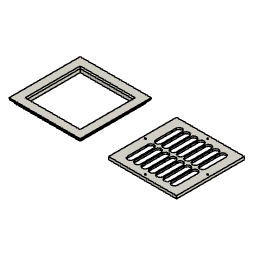
Magneto+Filter+Lüfter (Autodesk Fusion 360 design; units mm, degrees)
Autodesk Fusion 360 part; units mm, degrees
sketch "Skizze1" plane through (0, 0, 0) normal (0, 0, 1) x (1, 0, 0)
  line L0 (173.376542, 106.779405) -> (293.376542, 106.779405)
  line L1 (293.376542, 106.779405) -> (293.376542, -13.220595)
  line L2 (293.376542, -13.220595) -> (173.376542, -13.220595)
  line L3 (173.376542, -13.220595) -> (173.376542, 106.779405)
  line L4 (283.376542, -3.220595) -> (183.376542, -3.220595)
  line L5 (183.376542, -3.220595) -> (183.376542, 96.779405)
  line L6 (183.376542, 96.779405) -> (283.376542, 96.779405)
  line L7 (283.376542, 96.779405) -> (283.376542, -3.220595)
  line L8 (286.376542, -6.220595) -> (180.376542, -6.220595)
  line L9 (180.376542, -6.220595) -> (180.376542, 99.779405)
  line L10 (180.376542, 99.779405) -> (286.376542, 99.779405)
  line L11 (286.376542, 99.779405) -> (286.376542, -6.220595)
  circle A0 centre (233.376542, 103.279405) radius 1.5
  circle A1 centre (289.876542, 46.779405) radius 1.5
  circle A2 centre (176.876542, 46.779405) radius 1.5
  circle A3 centre (233.376542, -9.720595) radius 1.5
  circle A4 centre (423.376542, 103.279405) radius 1.5
  line L12 (483.376542, 106.779405) -> (483.376542, -13.220595)
  circle A5 centre (479.876542, 46.779405) radius 1.5
  line L13 (363.376542, 106.779405) -> (483.376542, 106.779405)
  circle A6 centre (366.876542, 46.779405) radius 1.5
  line L14 (363.376542, -13.220595) -> (363.376542, 106.779405)
  circle A7 centre (423.376542, -9.720595) radius 1.5
  line L15 (483.376542, -13.220595) -> (363.376542, -13.220595)
  line L16 (469.376542, 90.779405) -> (469.376542, 2.779405)
  line L17 (458.376542, 90.779405) -> (458.376542, 2.779405)
  arc A8 (469.376542, 90.779405) -> (458.376542, 90.779405) centre (463.876542, 90.779405) ccw
  arc A9 (458.376542, 2.779405) -> (469.376542, 2.779405) centre (463.876542, 2.779405) ccw
  line L18 (456.043208, 90.779405) -> (456.043208, 2.779405)
  arc A10 (456.043208, 90.779405) -> (445.043208, 90.779405) centre (450.543208, 90.779405) ccw
  line L19 (445.043208, 90.779405) -> (445.043208, 2.779405)
  arc A11 (445.043208, 2.779405) -> (456.043208, 2.779405) centre (450.543208, 2.779405) ccw
  line L20 (442.709875, 90.779405) -> (442.709875, 2.779405)
  arc A12 (442.709875, 90.779405) -> (431.709875, 90.779405) centre (437.209875, 90.779405) ccw
  line L21 (431.709875, 90.779405) -> (431.709875, 2.779405)
  arc A13 (431.709875, 2.779405) -> (442.709875, 2.779405) centre (437.209875, 2.779405) ccw
  line L22 (429.376542, 90.779405) -> (429.376542, 2.779405)
  arc A14 (429.376542, 90.779405) -> (418.376542, 90.779405) centre (423.876542, 90.779405) ccw
  line L23 (418.376542, 90.779405) -> (418.376542, 2.779405)
  arc A15 (418.376542, 2.779405) -> (429.376542, 2.779405) centre (423.876542, 2.779405) ccw
  line L24 (416.043208, 90.779405) -> (416.043208, 2.779405)
  arc A16 (416.043208, 90.779405) -> (405.043208, 90.779405) centre (410.543208, 90.779405) ccw
  line L25 (405.043208, 90.779405) -> (405.043208, 2.779405)
  arc A17 (405.043208, 2.779405) -> (416.043208, 2.779405) centre (410.543208, 2.779405) ccw
  line L26 (402.709875, 90.779405) -> (402.709875, 2.779405)
  arc A18 (402.709875, 90.779405) -> (391.709875, 90.779405) centre (397.209875, 90.779405) ccw
  line L27 (391.709875, 90.779405) -> (391.709875, 2.779405)
  arc A19 (391.709875, 2.779405) -> (402.709875, 2.779405) centre (397.209875, 2.779405) ccw
  line L28 (389.376542, 90.779405) -> (389.376542, 2.779405)
  arc A20 (389.376542, 90.779405) -> (378.376542, 90.779405) centre (383.876542, 90.779405) ccw
  line L29 (378.376542, 90.779405) -> (378.376542, 2.779405)
  arc A21 (378.376542, 2.779405) -> (389.376542, 2.779405) centre (383.876542, 2.779405) ccw
  dimension "d18" = 120
  dimension "d19" = 120
  dimension "d20" = 10
  dimension "d21" = 7
  dimension "d22" = 3
  dimension "d23" = 3
  dimension "d24" = 3
  dimension "d25" = 3
  dimension "d28" = 120
  dimension "d29" = 120
  dimension "d30" = 3
  dimension "d31" = 3
  dimension "d32" = 3
  dimension "d33" = 3
  dimension "d42" = -80
  dimension "d43" = 0
  constraint horizontal L0
  constraint vertical L1
  constraint horizontal L2
  constraint vertical L3
  constraint horizontal L13
  constraint vertical L12
  constraint horizontal L15
  constraint vertical L14
  constraint tangent L16 A9
  measures "d22" diameter of A0
  measures "d23" diameter of A1
  measures "d24" diameter of A2
  measures "d25" diameter of A3
  measures "d30" diameter of A4
  measures "d31" diameter of A5
  measures "d32" diameter of A6
  measures "d33" diameter of A7
extrude "Extrusion1" add sketch "Skizze1" along normal blind 10 contours L8 L9 L10 L11 picked at (216.709875, 98.779405) makes body 1
extrude "Extrusion2" add sketch "Skizze1" along normal blind 3 contours L0 L1 L2 L3 picked at (271.434124, -10.03234) bodies 1
extrude "Extrusion3" add sketch "Skizze1" along normal blind 3 separate body contours L12 L13 L14 L15 picked at (369.231464, 11.721823) makes body 2
sketch "Skizze2" plane through (0, 0, 10) normal (0, 0, 1) x (-1, 0, 0)
  line L0 (-183.376542, -96.779405) -> (-283.376542, -96.779405)
  line L1 (-283.376542, -96.779405) -> (-283.376542, 3.220595)
  line L2 (-283.376542, 3.220595) -> (-183.376542, 3.220595)
  line L3 (-183.376542, 3.220595) -> (-183.376542, -96.779405)
  line L4 (-286.376542, -99.779405) -> (-180.376542, -99.779405)
  line L5 (-180.376542, -99.779405) -> (-180.376542, 6.220595)
  line L6 (-180.376542, 6.220595) -> (-286.376542, 6.220595)
  line L7 (-286.376542, 6.220595) -> (-286.376542, -99.779405)
  line L8 (59.486834, 54.037754) -> (-90.513166, 54.037754)
  line L9 (-90.513166, 54.037754) -> (-90.513166, 204.037754)
  line L10 (-90.513166, 204.037754) -> (59.486834, 204.037754)
  line L11 (59.486834, 204.037754) -> (59.486834, 54.037754)
  line L12 (44.486834, 69.037754) -> (-75.513166, 69.037754)
  line L13 (-75.513166, 69.037754) -> (-75.513166, 189.037754)
  line L14 (-75.513166, 189.037754) -> (44.486834, 189.037754)
  line L15 (44.486834, 189.037754) -> (44.486834, 69.037754)
  dimension "d52" = 150
  dimension "d53" = 150
  dimension "d54" = 15
  constraint horizontal L8
  constraint vertical L9
  constraint horizontal L10
  constraint vertical L11
scale "Maßstab1" factor 1.2 about (283.376542, 96.779405, 0) bodies 1
scale "Maßstab2" factor 1.2 about (363.376542, 106.779405, 3) bodies 2
sketch "Skizze3" plane through (0, 0, 0) normal (0, 0, 1) x (1, 0, 0)
extrude "Extrusion4" add sketch "Skizze2" along normal blind 3 separate body contours L8 L9 L10 L11 picked at (-85.513166, 149.037754) makes body 3
move_body "Verschieben1" bodies 3 to x (1, 0, 0) y (0, 1, 0) z (0, 0, 1) at (207.863376, 165.817159, 2)
move_body "Verschieben2" bodies 3 to x (1, 0, 0) y (0, 1, 0) z (0, 0, 1) at (0, 0, -3)
move_body "Verschieben3" bodies 3 to x (1, 0, 0) y (0, 1, 0) z (0, 0, 1) at (0, 0, -1)
move_body "Verschieben4" bodies 3 to x (1, 0, 0) y (0, 1, 0) z (0, 0, 1) at (0, 0, -1)
extrude "Extrusion5" cut 1 faces at (203.376542, 99.179405, 12) along direction (0, 0, -1) blind 1 on bodies 1 bodies 1
extrude "Extrusion6" cut 1 faces at (203.376542, 99.179405, 11) along direction (0, 0, -1) blind 1 on bodies 1 bodies 1
combine "Kombinieren1" operation add target body 3 tool bodies 1
extrude "Extrusion7" add 1 faces at (155.202448, -8.889694, 3.6) along direction (0, 0, 1) blind 3.5 on bodies 3 bodies 3
sketch "Skizze4" plane through (0, 0, 3) normal (0, 0, 1) x (-1, 0, 0)
  arc A0 (-394.576542, -87.579405) -> (-381.376542, -87.579405) centre (-387.976542, -87.579405) ccw
  line L0 (-394.576542, -87.579405) -> (-394.576542, 18.020595)
  arc A1 (-381.376542, 18.020595) -> (-394.576542, 18.020595) centre (-387.976542, 18.020595) ccw
  line L1 (-381.376542, 18.020595) -> (-381.376542, -87.579405)
  circle A2 centre (-435.376542, 33.020595) radius 1.8
  arc A3 (-458.576542, -87.579405) -> (-445.376542, -87.579405) centre (-451.976542, -87.579405) ccw
  line L2 (-458.576542, -87.579405) -> (-458.576542, 18.020595)
  arc A4 (-445.376542, 18.020595) -> (-458.576542, 18.020595) centre (-451.976542, 18.020595) ccw
  line L3 (-445.376542, 18.020595) -> (-445.376542, -87.579405)
  arc A5 (-474.576542, -87.579405) -> (-461.376542, -87.579405) centre (-467.976542, -87.579405) ccw
  line L4 (-474.576542, -87.579405) -> (-474.576542, 18.020595)
  arc A6 (-461.376542, 18.020595) -> (-474.576542, 18.020595) centre (-467.976542, 18.020595) ccw
  line L5 (-461.376542, 18.020595) -> (-461.376542, -87.579405)
  arc A7 (-426.576542, -87.579405) -> (-413.376542, -87.579405) centre (-419.976542, -87.579405) ccw
  line L6 (-426.576542, -87.579405) -> (-426.576542, 18.020595)
  arc A8 (-413.376542, 18.020595) -> (-426.576542, 18.020595) centre (-419.976542, 18.020595) ccw
  line L7 (-413.376542, 18.020595) -> (-413.376542, -87.579405)
  circle A9 centre (-503.176542, -34.779405) radius 1.8
  arc A10 (-490.576542, -87.579405) -> (-477.376542, -87.579405) centre (-483.976542, -87.579405) ccw
  line L8 (-490.576542, -87.579405) -> (-490.576542, 18.020595)
  arc A11 (-477.376542, 18.020595) -> (-490.576542, 18.020595) centre (-483.976542, 18.020595) ccw
  line L9 (-477.376542, 18.020595) -> (-477.376542, -87.579405)
  arc A12 (-410.576542, -87.579405) -> (-397.376542, -87.579405) centre (-403.976542, -87.579405) ccw
  line L10 (-410.576542, -87.579405) -> (-410.576542, 18.020595)
  arc A13 (-397.376542, 18.020595) -> (-410.576542, 18.020595) centre (-403.976542, 18.020595) ccw
  line L11 (-397.376542, 18.020595) -> (-397.376542, -87.579405)
  circle A14 centre (-435.376542, -102.579405) radius 1.8
  circle A15 centre (-367.576542, -34.779405) radius 1.8
  arc A16 (-442.576542, -87.579405) -> (-429.376542, -87.579405) centre (-435.976542, -87.579405) ccw
  line L12 (-442.576542, -87.579405) -> (-442.576542, 18.020595)
  arc A17 (-429.376542, 18.020595) -> (-442.576542, 18.020595) centre (-435.976542, 18.020595) ccw
  line L13 (-429.376542, 18.020595) -> (-429.376542, -87.579405)
  line L14 (-507.376542, 37.220595) -> (-507.376542, -106.779405)
  line L15 (-507.376542, -106.779405) -> (-363.376542, -106.779405)
  line L16 (-363.376542, -106.779405) -> (-363.376542, 37.220595)
  line L17 (-363.376542, 37.220595) -> (-507.376542, 37.220595)
  line L18 (-509.376542, 39.220595) -> (-361.376542, 39.220595)
  line L19 (-361.376542, 39.220595) -> (-361.376542, -108.779405)
  line L20 (-361.376542, -108.779405) -> (-509.376542, -108.779405)
  line L21 (-509.376542, -108.779405) -> (-509.376542, 39.220595)
  line L22 (-363.376542, -106.779405) -> (-507.376542, -106.779405)
  line L23 (-507.376542, -106.779405) -> (-507.376542, 37.220595)
  line L24 (-507.376542, 37.220595) -> (-363.376542, 37.220595)
  line L25 (-363.376542, 37.220595) -> (-363.376542, -106.779405)
  constraint horizontal L18
  constraint vertical L19
  constraint horizontal L20
  constraint vertical L21
  constraint horizontal L22
  constraint vertical L23
  constraint horizontal L24
  constraint vertical L25
sketch "Skizze5" plane through (381.376542, 0, 0) normal (1, 0, 0) x (0, 1, 0)
  line L0 (-18.020595, -0.6) -> (87.579405, -0.6)
  line L1 (87.579405, -0.6) -> (87.579405, 3)
  line L2 (87.579405, 3) -> (-18.020595, 3)
  line L3 (-18.020595, 3) -> (-18.020595, -0.6)
  line L4 (87.579405, 3, 109.2) -> (-18.020595, 3, 109.2)
  line L5 (36.779405, 3, 0) -> (36.779405, 3, 109.2)
  line L6 (32.779405, 3, 0) -> (32.779405, 3, 109.2)
extrude "Extrusion8" add sketch "Skizze5" against normal blind 3.5 separate body contours L2 L4 L5 L6 in plane through (381.376542, 0, 3) normal (0, 0, 1) picked at (417.776542, 35.446072, 3) makes body 4
extrude "Extrusion9" add sketch "Skizze4" against normal blind 6 contours L18 L19 L20 L21 picked at (-508.709875, -10.779405) bodies 2
combine "Kombinieren2" operation add target body 2 tool bodies 4
fillet "Abrundung1" radius 6.6 6 edges at (394.576542, 36.779405, 1.25) (410.576542, 36.779405, 1.25) (426.576542, 36.779405, 1.25) (381.376542, 36.779405, 1.25) (397.376542, 36.779405, 1.25) (413.376542, 36.779405, 1.25) on bodies 2
fillet "Abrundung2" radius 6.6 8 edges at (442.576542, 36.779405, 1.25) (458.576542, 36.779405, 1.25) (474.576542, 36.779405, 1.25) (490.576542, 36.779405, 1.25) (429.376542, 36.779405, 1.25) (445.376542, 36.779405, 1.25) (461.376542, 36.779405, 1.25) (477.376542, 36.779405, 1.25) on bodies 2
fillet "Abrundung3" radius 6.6 14 edges at (490.576542, 32.779405, 1.25) (474.576542, 32.779405, 1.25) (458.576542, 32.779405, 1.25) (442.576542, 32.779405, 1.25) (426.576542, 32.779405, 1.25) (410.576542, 32.779405, 1.25) (394.576542, 32.779405, 1.25) (477.376542, 32.779405, 1.25) (461.376542, 32.779405, 1.25) (445.376542, 32.779405, 1.25) (429.376542, 32.779405, 1.25) (413.376542, 32.779405, 1.25) (397.376542, 32.779405, 1.25) (381.376542, 32.779405, 1.25) on bodies 2
sketch "Skizze6" plane through (0, 0, 0) normal (0, 0, 1) x (1, 0, 0)
  circle A0 centre (-185.976349, 60.387615) radius 2.5
  point P0 (-80.976349, 60.387615)
  point P1 (-185.976349, 165.387615)
  point P2 (-80.976349, 165.387615)
  dimension "d77" = 5
  dimension "d80" = 105
  dimension "d81" = 105
  measures "d77" diameter of A0
extrude "Extrusion10" add 1 faces at (163.376542, 16.779405, 6.666667) along direction (1, 0, 0) blind 2.5 on bodies 3 bodies 3
extrude "Extrusion11" add 1 faces at (205.043208, 96.779405, 3.333333) along direction (0, -1, 0) blind 2.5 on bodies 3 bodies 3
extrude "Extrusion12" add 1 faces at (283.376542, 55.112739, 3.333333) along direction (-1, 0, 0) blind 2.5 on bodies 3 bodies 3
extrude "Extrusion13" add 1 faces at (242.543208, -23.220595, 6.666667) along direction (0, 1, 0) blind 2.5 on bodies 3 bodies 3
chamfer "Fase1" distance 2.5 angle 45 4 edges at (165.876542, 36.779405, 10) (223.376542, 94.279405, 10) (280.876542, 36.779405, 10) (223.376542, -20.720595, 10) on bodies 3
extrude "Extrusion14" add 1 faces at (298.376542, 61.779405, 8) along direction (1, 0, 0) blind 2.5 on bodies 3 bodies 3
extrude "Extrusion15" add 1 faces at (250.043208, -38.220595, 8) along direction (0, -1, 0) blind 2.5 on bodies 3 bodies 3
extrude "Extrusion16" add 1 faces at (250.043208, 111.779405, 8) along direction (0, 1, 0) blind 2.5 on bodies 3 bodies 3
extrude "Extrusion17" add 1 faces at (148.376542, 62.612739, 8) along direction (-1, 0, 0) blind 2.5 on bodies 3 bodies 3
move_body "Verschieben5" bodies 2 to x (1, 0, 0) y (0, 1, 0) z (0, 0, 1) at (0, 0, 3)
